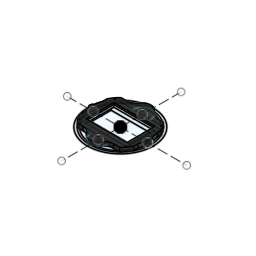
Glasträger v5 (Autodesk Fusion 360 design; units mm, degrees)
Autodesk Fusion 360 part; units mm, degrees
note: some values were not read from the file. Set by a fixed rule: which sketch regions a step uses; the direction of a hole.
sketch "Skizze1" plane through (0, 0, 0) normal (0, 0, 1) x (1, 0, 0)
  circle A0 centre (0, 0) radius 24.75
  circle A1 centre (0, 0) radius 21.75
  line L0 (-17.5, 13.5) -> (17.5, 13.5)
  line L1 (17.5, 13.5) -> (17.5, -13.5)
  line L2 (17.5, -13.5) -> (-17.5, -13.5)
  line L3 (-17.5, -13.5) -> (-17.5, 13.5)
  line L4 (-40, 0) -> (50, 0) construction
  line L5 (0, 45.7661) -> (0, -44.2339) construction
  line L6 (-16.0234, 16.5) -> (16.0234, 16.5)
  line L7 (20.5, 10.4283) -> (20.5, -10.4283)
  line L8 (16.0234, -16.5) -> (-16.0234, -16.5)
  line L9 (-20.5, -10.4283) -> (-20.5, 10.4283)
  arc A2 (6.5, 16.5) -> (-6.5, 16.5) centre (0, 16.5) ccw
  arc A3 (-6.6213, -16.5) -> (6.3787, -16.5) centre (-0.1213, -16.5) ccw
  arc A4 (-21.6357, 2.2272) -> (-21.6357, -2.2272) centre (-20.5, 0) ccw
  arc A5 (21.6357, -2.2272) -> (21.6357, 2.2272) centre (20.5, 0) ccw
  circle A6 centre (0, 0) radius 23
  line L10 (-14.5, -7.5) -> (14.5, -7.5)
  line L11 (14.5, -7.5) -> (14.5, 7.5)
  line L12 (14.5, 7.5) -> (-14.5, 7.5)
  line L13 (-14.5, 7.5) -> (-14.5, -7.5)
  line L14 (-15.5, 10.5) -> (15.5, 10.5)
  line L15 (15.5, 10.5) -> (15.5, -10.5)
  line L16 (15.5, -10.5) -> (-15.5, -10.5)
  line L17 (-15.5, -10.5) -> (-15.5, 10.5)
  dimension "d1" = 49.5
  dimension "d3" = 3
  dimension "d4" = 27
  dimension "d5" = 35
  dimension "d6" = 3
  dimension "d7" = 3
  dimension "d8" = 3
  dimension "d9" = 3
  dimension "d18" = 46
  dimension "d19" = 29
  dimension "d20" = 15
  dimension "d27" = 3
  dimension "d28" = 3
  dimension "d29" = 2
  dimension "d30" = 2
  dimension "d40" = 33
  constraint coincident A0.centre A1.centre
  constraint horizontal L0
  constraint vertical L1
  constraint horizontal L2
  constraint vertical L3
  constraint parallel L2 L4
  constraint symmetric L0 L2 L4
  constraint vertical L5
  constraint symmetric L1 L3 L5
  constraint coincident A0.centre L5
  constraint coincident A0.centre L4
  constraint horizontal L6
  constraint vertical L7
  constraint horizontal L8
  constraint vertical L9
  constraint equal A2 A3
  constraint coincident L6 A2.end
  constraint coincident L6 A2.start
  constraint coincident L8 A3.end
  constraint coincident L8 A3.start
  constraint coincident L8 A3.centre
  constraint coincident L6 A2.centre
  constraint equal A4 A5
  constraint coincident A1 A4.start
  constraint coincident A1 A4.end
  constraint concentric A0 A6
  constraint tangent A5 A6
  constraint tangent A2 A6
  constraint horizontal L10
  constraint vertical L11
  constraint horizontal L12
  constraint vertical L13
  constraint symmetric L5 L11 L13
  constraint symmetric L4 L10 L12
  constraint coincident A6 L7.end
  constraint coincident L7 A5.centre
  constraint coincident A6 L8.start
  constraint coincident A6 L9.start
  constraint coincident L9 A4.centre
  constraint coincident A6 L8.end
  constraint coincident A6 L6.start
  constraint coincident A6 L9.end
  constraint coincident A6 L6.end
  constraint coincident A6 L7.start
  constraint coincident A1 A5.end
  constraint coincident A1 A5.start
  constraint horizontal L14
  constraint vertical L15
  constraint horizontal L16
  constraint vertical L17
  measures "d1" diameter of A0
  measures "d3" distance of A0 A1
  measures "d4" distance of L0.start L2.end
  measures "d5" distance of L0.start L0.end
  measures "d6" distance of L3 L9
  measures "d7" distance of L1 L7
  measures "d8" distance of L0 L6
  measures "d9" distance of L2 L8
  measures "d18" diameter of A6
  measures "d19" distance of L10.start L10.end
  measures "d20" distance of L10.end L11.end
  measures "d27" distance of L0 L14
  measures "d28" distance of L2 L16
  measures "d29" distance of L1 L15
  measures "d30" distance of L3 L17
  measures "d40" distance of L6 L8
extrude "Extrusion5" add sketch "Skizze1" along normal blind 3 contours A1 L7 | A1 A5 | A1 L1 L7 | A1 L0 L1 L6 L7 A6 | A1 L1 L2 L7 L8 A6 | A1 L0 L6 | A1 L2 L8 | A1 L0 L3 L6 L9 A6 | A1 A2 | A1 A3 | A1 L2 L3 L8 L9 A6 | A1 L6 A2 | A1 L3 L9 | A1 L8 A3 | A1 L9 | A1 A4 picked at (0.4894, 18.2335) picked at (-0.6234, -18.2297)
extrude "Extrusion6" add sketch "Skizze1" along normal up to surface (1.5 mm away) from surface at 1.5 contours A1 L0 L1 L2 L3
hole "Bohrung1" at (0, 16.5, 0) at (20.5, 0, 0) at (-0.1213, -16.5, 0) at (-20.5, 0, 0) direction (0, 0, 1) diameter 2.5 end through all
fillet "Abrundung1" radius 7 4 edges at (-6.6213, -16.5, 1.5) (6.3787, -16.5, 1.5) (6.5, 16.5, 1.5) (-6.5, 16.5, 1.5)
